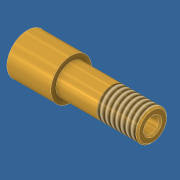
# Autodesk Inventor part: SlipRingExtender
Saved by Autodesk Inventor 2016 (Build 200138000, 138)
## iProperties
Created: 2016-03-29
Part Number: SlipRingExtender
Material: Messing, weicher Gelbton
Document SubType Name: Modeling
Designer: 4ndreas
Density: 8.47 g/cm^3
Appearance: Messing - satiniert
Mass: 5.55451 g
Surface Area: 8.52573 cm^2
Volume: 0.655787 cm^3
Author: 4ndreas
Autodesk Inventor part; units mm, degrees
ref_plane "YZ Plane" through (0, 0, 0) normal (1, 0, 0) x (0, 1, 0)
ref_plane "XZ Plane" through (0, 0, 0) normal (0, 1, 0) x (-1, 0, 0)
ref_plane "XY Plane" through (0, 0, 0) normal (0, 0, 1) x (1, 0, 0)
sketch "Skizze1" plane through (0, 0, 0) normal (0, 0, 1) x (1, 0, 0)
  line L0 (0, 0) -> (24.6, 0)
  line L1 (0, 0) -> (0, 4)
  line L2 (0, 4) -> (8.6, 4)
  line L3 (8.6, 4) -> (8.6, 3)
  line L4 (8.6, 3) -> (24.6, 3)
  line L5 (24.6, 3) -> (24.6, 0)
  dimension "d0" = 8
  dimension "d1" = 6
  dimension "d2" = 8.6
  dimension "d3" = 16
  constraints: 12 end point, 4 perpendicular, 1 horizontal, 1 vertical
  measures "d0" diameter of L2 L0
  measures "d1" diameter of L4 L0
  measures "d2" distance between parallel lines of L1 L3
  measures "d3" distance between parallel lines of L3 L5
revolve "Umdrehung1" add sketch "Skizze1" angle 360 about axis through (0, 0, 0) along (1, 0, 0)
sketch "Skizze2" plane through (0, 0, 0) normal (-1, 0, 0) x (0, 0, 1)
  point P0 (0, 0)
hole "Bohrung1" at (0, 0, 0) direction (1, 0, 0) diameter 3 end through all
hole "Bohrung2" at (0, 0, 0) direction (1, 0, 0) diameter 5 depth 4 tip angle 118
thread "Gewinde1" size "M6x1" class "6g" standard "ANSI Metric M Profile" length 8
chamfer "Fase1" distance 0.3 angle 45 2 edges at (24.6, -3, 0) (24.6, 0, -1.5)
